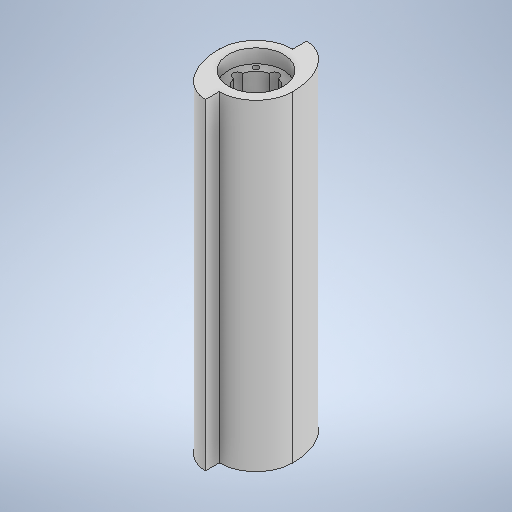
# Autodesk Inventor part: Барабан
Saved by Autodesk Inventor 2025.1 (Build 291241000, 241)
## iProperties
Created: 2025-04-10
Part Number: Барабан
Material: Типовые
Document SubType Name: Modeling
Designer: tishk
Density: 1 g/cm^3
Appearance: По умолчанию
Author: tishk
Autodesk Inventor part; units mm, degrees
ref_plane "YZ Plane" through (0, 0, 0) normal (1, 0, 0) x (0, 1, 0)
ref_plane "XZ Plane" through (0, 0, 0) normal (0, 1, 0) x (-1, 0, 0)
ref_plane "XY Plane" through (0, 0, 0) normal (0, 0, 1) x (1, 0, 0)
sketch "Эскиз1" plane through (0, 0, 0) normal (0, 1, 0) x (-1, 0, 0)
  circle A0 centre (0, 0) radius 20
  ellipse E0 centre (0, 0) end of major axis (0, -55) minor radius 40 (40, 0) -> (0, 55) ccw
  ellipse E1 centre (0, 0) end of major axis (0, -55) minor radius 40 (-40, 0) -> (0, -55) ccw
  arc A1 (0, -40) -> (40, 0) centre (0, 0) ccw
  arc A2 (0, 40) -> (-40, 0) centre (0, 0) ccw
  line L0 (0, 55) -> (0, 40)
  line L1 (0, -40) -> (0, -55)
  line L2 (0, -40) -> (0, -55)
  line L3 (0, 40) -> (0, 55)
  dimension "d0" = 40
  dimension "d2" = 55
  dimension "d3" = 55
  constraints: 8 end point, 4 point on circle, 3 centre point, 3 coincident, 3 vertical, 1 collinear, 8 other
  measures "d0" diameter of A0
  measures "d2" distance of A1.centre L1.end
  measures "d3" distance of A1.centre L0.start
extrude "Выдавливание1" add sketch "Эскиз1" along normal blind 350
sketch "Эскиз2" plane through (0, 350, 0) normal (0, 1, 0) x (1, 0, 0)
  point P0 (0, 0)
hole "Отверстие1" at (0, 350, 0) direction (0, -1, 0) diameter 60 depth 15
sketch "Эскиз3" plane through (0, 350, 0) normal (0, 1, 0) x (1, 0, 0)
  line L0 (0, 0) -> (-20, 0)
  circle A0 centre (0, 0) radius 20 projected
  line L1 (0, 0) -> (0, 20)
  line L2 (0, 0) -> (0, -20)
  line L3 (0, 0) -> (20, 0)
  constraints: 8 end point, 4 point on circle, 2 perpendicular, 1 horizontal, 1 vertical
hole "Отверстие2" at (-20, 350, 0) at (0, 350, -20) at (20, 350, 0) at (0, 350, 20) direction (0, -1, 0) diameter 10 depth 45
sketch "Эскиз4" plane through (0, 0, 0) normal (0, -1, 0) x (1, 0, 0)
  circle A0 centre (0, 0) radius 30
  constraints: 1 centre point, 1 coincident
hole "Отверстие3" at (0, 0, 0) direction (0, 1, 0) diameter 60 depth 15
sketch "Эскиз5" plane through (0, 0, 0) normal (0, -1, 0) x (1, 0, 0)
  line L0 (0, 0) -> (-14.1421, -14.1421)
  line L1 (0, 0) -> (20, 0) construction
  line L2 (0, 0) -> (-14.1421, 14.1421)
  arc A0 (-4.9608, 19.375) -> (-19.375, 4.9608) centre (0, 0) ccw projected
  line L3 (0, 0) -> (14.1421, 14.1421)
  line L4 (0, 0) -> (14.1421, -14.1421)
  dimension "d27" = 20
  dimension "d28" = 135
  constraints: 10 end point, 1 equal length, 1 horizontal, 1 perpendicular, 1 point on circle
  measures "d27" distance of L0.start L0.end
  measures "d28" angle of L0 L1
hole "Отверстие4" at (14.1421, 0, -14.1421) at (-14.1421, 0, 14.1421) at (14.1421, 0, 14.1421) at (-14.1421, 0, -14.1421) direction (0, 1, 0) diameter 10 depth 45
sketch "Эскиз6" plane through (0, 0, 0) normal (0, -1, 0) x (1, 0, 0)
  line L0 (0, 0) -> (0, 25)
  arc A0 (4.9608, 19.375) -> (-4.9608, 19.375) centre (0, 20) ccw projected
  line L1 (0, 0) -> (-25, 0)
  arc A1 (-19.375, 4.9608) -> (-19.375, -4.9608) centre (-20, 0) ccw projected
  line L2 (0, 0) -> (0, -25)
  arc A2 (-4.9608, -19.375) -> (4.9608, -19.375) centre (0, -20) ccw projected
  line L3 (0, 0) -> (25, 0)
  arc A3 (19.375, -4.9608) -> (19.375, 4.9608) centre (20, 0) ccw projected
  constraints: 8 end point, 4 point on circle, 2 vertical, 1 horizontal, 1 perpendicular
hole "Отверстие5" at (0, 0, -25) at (-25, 0, 0) at (0, 0, 25) at (25, 0, 0) direction (0, 1, 0) diameter 6 depth 25
sketch "Эскиз7" plane through (0, 350, 0) normal (0, 1, 0) x (1, 0, 0)
  line L0 (0, 0) -> (-17.6771, 17.6782)
  arc A0 (-10.1924, 17.208) -> (-17.208, 10.1924) centre (-14.1421, 14.1421) ccw projected
  line L1 (0, 0) -> (-17.6782, -17.6771)
  arc A1 (-17.208, -10.1924) -> (-10.1924, -17.208) centre (-14.1421, -14.1421) ccw projected
  line L2 (0, 0) -> (17.6771, -17.6782)
  arc A2 (10.1924, -17.208) -> (17.208, -10.1924) centre (14.1421, -14.1421) ccw projected
  line L3 (0, 0) -> (17.6782, 17.6771)
  arc A3 (17.208, 10.1924) -> (10.1924, 17.208) centre (14.1421, 14.1421) ccw projected
  constraints: 8 end point, 4 point on circle, 2 point on line, 1 perpendicular
hole "Отверстие6" at (-17.6782, 350, 17.6771) at (-17.6771, 350, -17.6782) at (17.6782, 350, -17.6771) at (17.6771, 350, 17.6782) direction (0, -1, 0) diameter 6 depth 25
